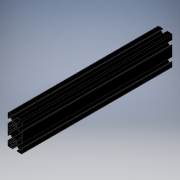
# Autodesk Inventor part: 20-2040-Black-203.2-CL
Saved by Autodesk Inventor 2019 (Build 230136000, 136)
## iProperties
Created: 2022-06-30
Part Number: 20-2040-Black-203.2-CL
Material: Generic
Catalog Web Link: www.cadenas.de
Description: 20-2040, 20-2040-Black-T-Slotted Profile - 20 Series
Vendor: 8020
Document SubType Name: Modeling
Designer: psAdmin
Manufacturer: 8020
Mass: 55.9614 g
Surface Area: 682.674 cm^2
Volume: 55.9614 cm^3
Density: 1 g/cm^3
Appearance: PSOLRGB-0-0-0
Category: PARTsolutions
Company: 8020
Title: 20-2040-Black-203.2
Author: Cadenas PARTsolutions
Comments: T-Slotted Profile - 20 Series
PSOL_IDENT_0: {$CADENAS_DATA/23d-libs/8020/metric/profiles/20_series/20_2040.prj},206 {VTYP=3D},{NB=20-2040-Black-
PSOL_IDENT_1: 203.2-CL},{LINA=20-2040-Black-203.2},{NN=20-2040, 20-2040-Black},{DATE=31.07.2020 09:21:32},{GEOMDAT
PSOL_IDENT_2: E=09.02.2018 15:35:30},{VERSION=},{LINEID=10},{WBVAR=FIN,LS,L},{WBNUMERIC=L}  {NB=20-2040-Black-203.
PSOL_IDENT_3: 2-CL},{LINA=20-2040-Black-203.2},{KT=DUMMY},{PN=20-2040-Black-203.2},{PN1=20-2040},{FIN=BA},{LS=-CL}
PSOL_IDENT_4: ,{L=203.20},{SERIES=20-2040},{MAT=6105-T5 Aluminum},{W=0.7649},{LALG=[25:6000/0.05]},{MIX=4.5357},{M
PSOL_IDENT_5: IY=1.2133},{EA=2.7467},{COLOR=0,0,0}
NB: 20-2040-Black-203.2-CL
NN: 20-2040, 20-2040-Black
NT: T-Slotted Profile - 20 Series
NBSYN: $PN.$LS.
LINA: 20-2040-Black-203.2
CATALOG: 80/20
PN: 20-2040-Black-203.2
FIN: Black Anodize
LS: Custom Length
L: 203.2
SERIES: 20-2040
MAT: 6105-T5 Aluminum
W: 0.7649
MIX: 4.5357
MIY: 1.2133
EA: 2.7467
SUPPLIER: 8020
ARTICLENO: 20-2040-Black-203.2-CL
BOMINFO: 20-2040-Black-203.2
CREATOR: CADENAS GmbH
Autodesk Inventor part; units mm, degrees
ref_plane "YZ Plane" through (0, 0, 0) normal (1, 0, 0) x (0, 1, 0)
ref_plane "XZ Plane" through (0, 0, 0) normal (0, 1, 0) x (-1, 0, 0)
ref_plane "XY Plane" through (0, 0, 0) normal (0, 0, 1) x (1, 0, 0)
sketch "Sketch_1" plane through (0, 0, 0) normal (0, 0, 1) x (1, 0, 0)
  line L0 (-10, 28.5) -> (-10, 23.138)
  arc A0 (-10, 23.138) -> (-9.492, 22.63) centre (-9.492, 23.138) ccw
  line L1 (-9.492, 22.63) -> (-9.008, 22.63)
  arc A1 (-9.008, 22.63) -> (-8.5, 23.138) centre (-9.008, 23.138) ccw
  line L2 (-8.5, 23.138) -> (-8.5, 25.487)
  arc A2 (-7.992, 25.995) -> (-8.5, 25.487) centre (-7.992, 25.487) ccw
  line L3 (-7.992, 25.995) -> (-7.2659, 25.995)
  arc A3 (-6.9067, 25.8462) -> (-7.2659, 25.995) centre (-7.2659, 25.487) ccw
  line L4 (-6.9067, 25.8462) -> (-3.8038, 22.7433)
  arc A4 (-3.655, 22.3841) -> (-3.8038, 22.7433) centre (-4.163, 22.3841) ccw
  line L5 (-3.655, 22.3841) -> (-3.655, 17.6162)
  arc A5 (-3.8038, 17.257) -> (-3.655, 17.6162) centre (-4.163, 17.6162) ccw
  line L6 (-3.8038, 17.257) -> (-6.907, 14.1538)
  arc A6 (-7.2662, 14.005) -> (-6.907, 14.1538) centre (-7.2662, 14.513) ccw
  line L7 (-7.2662, 14.005) -> (-7.992, 14.005)
  arc A7 (-8.5, 14.513) -> (-7.992, 14.005) centre (-7.992, 14.513) ccw
  line L8 (-8.5, 14.513) -> (-8.5, 16.862)
  arc A8 (-8.5, 16.862) -> (-9.008, 17.37) centre (-9.008, 16.862) ccw
  line L9 (-9.008, 17.37) -> (-9.492, 17.37)
  arc A9 (-9.492, 17.37) -> (-10, 16.862) centre (-9.492, 16.862) ccw
  line L10 (-10, 16.862) -> (-10, 3.138)
  arc A10 (-10, 3.138) -> (-9.492, 2.63) centre (-9.492, 3.138) ccw
  line L11 (-9.492, 2.63) -> (-9.008, 2.63)
  arc A11 (-9.008, 2.63) -> (-8.5, 3.138) centre (-9.008, 3.138) ccw
  line L12 (-8.5, 3.138) -> (-8.5, 5.487)
  arc A12 (-7.992, 5.995) -> (-8.5, 5.487) centre (-7.992, 5.487) ccw
  line L13 (-7.992, 5.995) -> (-7.2662, 5.995)
  arc A13 (-6.907, 5.8462) -> (-7.2662, 5.995) centre (-7.2662, 5.487) ccw
  line L14 (-6.907, 5.8462) -> (-3.8038, 2.743)
  arc A14 (-3.655, 2.3838) -> (-3.8038, 2.743) centre (-4.163, 2.3838) ccw
  line L15 (-3.655, 2.3838) -> (-3.655, -2.3841)
  arc A15 (-3.8038, -2.7433) -> (-3.655, -2.3841) centre (-4.163, -2.3841) ccw
  line L16 (-3.8038, -2.7433) -> (-6.9067, -5.8462)
  arc A16 (-7.2659, -5.995) -> (-6.9067, -5.8462) centre (-7.2659, -5.487) ccw
  line L17 (-7.2659, -5.995) -> (-7.992, -5.995)
  arc A17 (-8.5, -5.487) -> (-7.992, -5.995) centre (-7.992, -5.487) ccw
  line L18 (-8.5, -5.487) -> (-8.5, -3.138)
  arc A18 (-8.5, -3.138) -> (-9.008, -2.63) centre (-9.008, -3.138) ccw
  line L19 (-9.008, -2.63) -> (-9.492, -2.63)
  arc A19 (-9.492, -2.63) -> (-10, -3.138) centre (-9.492, -3.138) ccw
  line L20 (-10, -3.138) -> (-10, -8.5)
  arc A20 (-10, -8.5) -> (-8.5, -10) centre (-8.5, -8.5) ccw
  line L21 (-8.5, -10) -> (-3.138, -10)
  arc A21 (-3.138, -10) -> (-2.63, -9.492) centre (-3.138, -9.492) ccw
  line L22 (-2.63, -9.492) -> (-2.63, -9.008)
  arc A22 (-2.63, -9.008) -> (-3.138, -8.5) centre (-3.138, -9.008) ccw
  line L23 (-3.138, -8.5) -> (-5.487, -8.5)
  arc A23 (-5.995, -7.992) -> (-5.487, -8.5) centre (-5.487, -7.992) ccw
  line L24 (-5.995, -7.992) -> (-5.995, -7.2662)
  arc A24 (-5.8462, -6.907) -> (-5.995, -7.2662) centre (-5.487, -7.2662) ccw
  line L25 (-5.8462, -6.907) -> (-2.743, -3.8038)
  arc A25 (-2.3838, -3.655) -> (-2.743, -3.8038) centre (-2.3838, -4.163) ccw
  line L26 (-2.3838, -3.655) -> (2.3841, -3.655)
  arc A26 (2.7433, -3.8038) -> (2.3841, -3.655) centre (2.3841, -4.163) ccw
  line L27 (2.7433, -3.8038) -> (5.8462, -6.9067)
  arc A27 (5.995, -7.2659) -> (5.8462, -6.9067) centre (5.487, -7.2659) ccw
  line L28 (5.995, -7.2659) -> (5.995, -7.992)
  arc A28 (5.487, -8.5) -> (5.995, -7.992) centre (5.487, -7.992) ccw
  line L29 (5.487, -8.5) -> (3.138, -8.5)
  arc A29 (3.138, -8.5) -> (2.63, -9.008) centre (3.138, -9.008) ccw
  line L30 (2.63, -9.008) -> (2.63, -9.492)
  arc A30 (2.63, -9.492) -> (3.138, -10) centre (3.138, -9.492) ccw
  line L31 (3.138, -10) -> (8.5, -10)
  arc A31 (8.5, -10) -> (10, -8.5) centre (8.5, -8.5) ccw
  line L32 (10, -8.5) -> (10, -3.138)
  arc A32 (10, -3.138) -> (9.492, -2.63) centre (9.492, -3.138) ccw
  line L33 (9.492, -2.63) -> (9.008, -2.63)
  arc A33 (9.008, -2.63) -> (8.5, -3.138) centre (9.008, -3.138) ccw
  line L34 (8.5, -3.138) -> (8.5, -5.487)
  arc A34 (7.992, -5.995) -> (8.5, -5.487) centre (7.992, -5.487) ccw
  line L35 (7.992, -5.995) -> (7.2662, -5.995)
  arc A35 (6.907, -5.8462) -> (7.2662, -5.995) centre (7.2662, -5.487) ccw
  line L36 (6.907, -5.8462) -> (3.8038, -2.743)
  arc A36 (3.655, -2.3838) -> (3.8038, -2.743) centre (4.163, -2.3838) ccw
  line L37 (3.655, -2.3838) -> (3.655, 2.3841)
  arc A37 (3.8038, 2.7433) -> (3.655, 2.3841) centre (4.163, 2.3841) ccw
  line L38 (3.8038, 2.7433) -> (6.9067, 5.8462)
  arc A38 (7.2659, 5.995) -> (6.9067, 5.8462) centre (7.2659, 5.487) ccw
  line L39 (7.2659, 5.995) -> (7.992, 5.995)
  arc A39 (8.5, 5.487) -> (7.992, 5.995) centre (7.992, 5.487) ccw
  line L40 (8.5, 5.487) -> (8.5, 3.138)
  arc A40 (8.5, 3.138) -> (9.008, 2.63) centre (9.008, 3.138) ccw
  line L41 (9.008, 2.63) -> (9.492, 2.63)
  arc A41 (9.492, 2.63) -> (10, 3.138) centre (9.492, 3.138) ccw
  line L42 (10, 3.138) -> (10, 16.862)
  arc A42 (10, 16.862) -> (9.492, 17.37) centre (9.492, 16.862) ccw
  line L43 (9.492, 17.37) -> (9.008, 17.37)
  arc A43 (9.008, 17.37) -> (8.5, 16.862) centre (9.008, 16.862) ccw
  line L44 (8.5, 16.862) -> (8.5, 14.513)
  arc A44 (7.992, 14.005) -> (8.5, 14.513) centre (7.992, 14.513) ccw
  line L45 (7.992, 14.005) -> (7.2659, 14.005)
  arc A45 (6.9067, 14.1538) -> (7.2659, 14.005) centre (7.2659, 14.513) ccw
  line L46 (6.9067, 14.1538) -> (3.8038, 17.2567)
  arc A46 (3.655, 17.6159) -> (3.8038, 17.2567) centre (4.163, 17.6159) ccw
  line L47 (3.655, 17.6159) -> (3.655, 22.3838)
  arc A47 (3.8038, 22.743) -> (3.655, 22.3838) centre (4.163, 22.3838) ccw
  line L48 (3.8038, 22.743) -> (6.907, 25.8462)
  arc A48 (7.2662, 25.995) -> (6.907, 25.8462) centre (7.2662, 25.487) ccw
  line L49 (7.2662, 25.995) -> (7.992, 25.995)
  arc A49 (8.5, 25.487) -> (7.992, 25.995) centre (7.992, 25.487) ccw
  line L50 (8.5, 25.487) -> (8.5, 23.138)
  arc A50 (8.5, 23.138) -> (9.008, 22.63) centre (9.008, 23.138) ccw
  line L51 (9.008, 22.63) -> (9.492, 22.63)
  arc A51 (9.492, 22.63) -> (10, 23.138) centre (9.492, 23.138) ccw
  line L52 (10, 23.138) -> (10, 28.5)
  arc A52 (10, 28.5) -> (8.5, 30) centre (8.5, 28.5) ccw
  line L53 (8.5, 30) -> (3.138, 30)
  arc A53 (3.138, 30) -> (2.63, 29.492) centre (3.138, 29.492) ccw
  line L54 (2.63, 29.492) -> (2.63, 29.008)
  arc A54 (2.63, 29.008) -> (3.138, 28.5) centre (3.138, 29.008) ccw
  line L55 (3.138, 28.5) -> (5.487, 28.5)
  arc A55 (5.995, 27.992) -> (5.487, 28.5) centre (5.487, 27.992) ccw
  line L56 (5.995, 27.992) -> (5.995, 27.2659)
  arc A56 (5.8462, 26.9067) -> (5.995, 27.2659) centre (5.487, 27.2659) ccw
  line L57 (5.8462, 26.9067) -> (2.7433, 23.8038)
  arc A57 (2.3841, 23.655) -> (2.7433, 23.8038) centre (2.3841, 24.163) ccw
  line L58 (2.3841, 23.655) -> (-2.3838, 23.655)
  arc A58 (-2.743, 23.8038) -> (-2.3838, 23.655) centre (-2.3838, 24.163) ccw
  line L59 (-2.743, 23.8038) -> (-5.8462, 26.907)
  arc A59 (-5.995, 27.2662) -> (-5.8462, 26.907) centre (-5.487, 27.2662) ccw
  line L60 (-5.995, 27.2662) -> (-5.995, 27.992)
  arc A60 (-5.487, 28.5) -> (-5.995, 27.992) centre (-5.487, 27.992) ccw
  line L61 (-5.487, 28.5) -> (-3.138, 28.5)
  arc A61 (-3.138, 28.5) -> (-2.63, 29.008) centre (-3.138, 29.008) ccw
  line L62 (-2.63, 29.008) -> (-2.63, 29.492)
  arc A62 (-2.63, 29.492) -> (-3.138, 30) centre (-3.138, 29.492) ccw
  line L63 (-3.138, 30) -> (-8.5, 30)
  arc A63 (-8.5, 30) -> (-10, 28.5) centre (-8.5, 28.5) ccw
  arc A64 (-1.9358, -0.8037) -> (-2.3045, -2.1245) centre (-1.748, -1.568) ccw
  line L64 (-2.3045, -2.1245) -> (-2.1245, -2.3045)
  arc A65 (-2.1245, -2.3045) -> (-0.8037, -1.9358) centre (-1.568, -1.748) ccw
  arc A66 (-0.8037, -1.9358) -> (0.8037, -1.9358) centre (0, 0) ccw
  arc A67 (0.8037, -1.9358) -> (2.1245, -2.3045) centre (1.568, -1.748) ccw
  line L65 (2.1245, -2.3045) -> (2.3045, -2.1245)
  arc A68 (2.3045, -2.1245) -> (1.9358, -0.8037) centre (1.748, -1.568) ccw
  arc A69 (1.9358, -0.8037) -> (1.9358, 0.8037) centre (0, 0) ccw
  arc A70 (1.9358, 0.8037) -> (2.3045, 2.1245) centre (1.748, 1.568) ccw
  line L66 (2.3045, 2.1245) -> (2.1245, 2.3045)
  arc A71 (2.1245, 2.3045) -> (0.8037, 1.9358) centre (1.568, 1.748) ccw
  arc A72 (0.8037, 1.9358) -> (-0.8037, 1.9358) centre (0, 0) ccw
  arc A73 (-0.8037, 1.9358) -> (-2.1245, 2.3045) centre (-1.568, 1.748) ccw
  line L67 (-2.1245, 2.3045) -> (-2.3045, 2.1245)
  arc A74 (-2.3045, 2.1245) -> (-1.9358, 0.8037) centre (-1.748, 1.568) ccw
  arc A75 (-1.9358, 0.8037) -> (-1.9358, -0.8037) centre (0, 0) ccw
  arc A76 (-2.3045, 22.1245) -> (-1.9358, 20.8037) centre (-1.748, 21.568) ccw
  arc A77 (-1.9358, 20.8037) -> (-1.9358, 19.1963) centre (0, 20) ccw
  arc A78 (-1.9358, 19.1963) -> (-2.3045, 17.8755) centre (-1.748, 18.432) ccw
  line L68 (-2.3045, 17.8755) -> (-2.1245, 17.6955)
  arc A79 (-2.1245, 17.6955) -> (-0.8037, 18.0642) centre (-1.568, 18.252) ccw
  arc A80 (-0.8037, 18.0642) -> (0.8037, 18.0642) centre (0, 20) ccw
  arc A81 (0.8037, 18.0642) -> (2.1245, 17.6955) centre (1.568, 18.252) ccw
  line L69 (2.1245, 17.6955) -> (2.3045, 17.8755)
  arc A82 (2.3045, 17.8755) -> (1.9358, 19.1963) centre (1.748, 18.432) ccw
  arc A83 (1.9358, 19.1963) -> (1.9358, 20.8037) centre (0, 20) ccw
  arc A84 (1.9358, 20.8037) -> (2.3045, 22.1245) centre (1.748, 21.568) ccw
  line L70 (2.3045, 22.1245) -> (2.1245, 22.3045)
  arc A85 (2.1245, 22.3045) -> (0.8037, 21.9358) centre (1.568, 21.748) ccw
  arc A86 (0.8037, 21.9358) -> (-0.8037, 21.9358) centre (0, 20) ccw
  arc A87 (-0.8037, 21.9358) -> (-2.1245, 22.3045) centre (-1.568, 21.748) ccw
  line L71 (-2.1245, 22.3045) -> (-2.3045, 22.1245)
  arc A88 (-8.5, 8.003) -> (-7.992, 7.495) centre (-7.992, 8.003) ccw
  line L72 (-7.992, 7.495) -> (-6.6449, 7.495)
  arc A89 (-6.2857, 7.3462) -> (-6.6449, 7.495) centre (-6.6449, 6.987) ccw
  line L73 (-6.2857, 7.3462) -> (-2.7433, 3.8038)
  arc A90 (-2.7433, 3.8038) -> (-2.3841, 3.655) centre (-2.3841, 4.163) ccw
  line L74 (-2.3841, 3.655) -> (2.3838, 3.655)
  arc A91 (2.3838, 3.655) -> (2.743, 3.8038) centre (2.3838, 4.163) ccw
  line L75 (2.743, 3.8038) -> (6.2854, 7.3462)
  arc A92 (6.6446, 7.495) -> (6.2854, 7.3462) centre (6.6446, 6.987) ccw
  line L76 (6.6446, 7.495) -> (7.992, 7.495)
  arc A93 (7.992, 7.495) -> (8.5, 8.003) centre (7.992, 8.003) ccw
  line L77 (8.5, 8.003) -> (8.5, 11.997)
  arc A94 (8.5, 11.997) -> (7.992, 12.505) centre (7.992, 11.997) ccw
  line L78 (7.992, 12.505) -> (6.6446, 12.505)
  arc A95 (6.2854, 12.6538) -> (6.6446, 12.505) centre (6.6446, 13.013) ccw
  line L79 (6.2854, 12.6538) -> (2.743, 16.1962)
  arc A96 (2.743, 16.1962) -> (2.3838, 16.345) centre (2.3838, 15.837) ccw
  line L80 (2.3838, 16.345) -> (-2.3841, 16.345)
  arc A97 (-2.3841, 16.345) -> (-2.7433, 16.1962) centre (-2.3841, 15.837) ccw
  line L81 (-2.7433, 16.1962) -> (-6.2857, 12.6538)
  arc A98 (-6.6449, 12.505) -> (-6.2857, 12.6538) centre (-6.6449, 13.013) ccw
  line L82 (-6.6449, 12.505) -> (-7.992, 12.505)
  arc A99 (-7.992, 12.505) -> (-8.5, 11.997) centre (-7.992, 11.997) ccw
  line L83 (-8.5, 11.997) -> (-8.5, 8.003)
  constraints: 200 point on circle, 168 end point, 100 centre point
extrude "Extrusion1" add sketch "Sketch_1" against normal blind 203.2
body "Solid1"
